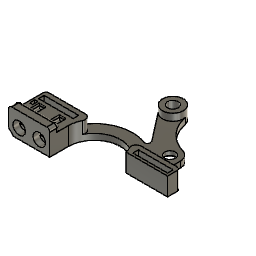
D_Prpbe_Mount v6 (Autodesk Fusion 360 design; units mm, degrees)
Autodesk Fusion 360 part; units mm, degrees
sketch "스케치1" plane through (0, 0, 0) normal (0, 0, 1) x (1, 0, 0)
  circle A0 centre (0, 0) radius 3.675
  circle A1 centre (17.5, -18.9) radius 3.675
  line L0 (30.625, -30.525) -> (30.625, -33.275)
  line L1 (30.625, -33.275) -> (13.375, -33.275)
  line L2 (13.375, -33.275) -> (13.375, -30.525)
  line L3 (-33.625, -33.275) -> (-16.375, -33.275)
  line L4 (-16.375, -33.275) -> (-16.375, -30.525)
  line L5 (-33.625, -30.525) -> (-33.625, -33.275)
  line L6 (-35, -28.225) -> (-18.0402, -28.225)
  line L7 (-14.55, -37.575) -> (-14.55, -46.814)
  line L8 (-14.55, -46.814) -> (-35, -46.814)
  line L9 (-35, -46.814) -> (-35, -28.225)
  line L10 (22.675, -28.225) -> (31.925, -28.225)
  line L11 (31.925, -28.225) -> (31.925, -34.575)
  line L12 (31.925, -34.575) -> (11.2005, -34.575)
  line L13 (22.675, -18.9) -> (22.675, -28.225)
  arc A2 (5.0614, 1.0785) -> (18.9641, -13.9364) centre (24.6222, 5.2465) ccw
  arc A3 (22.675, -18.9) -> (18.9641, -13.9364) centre (17.5, -18.9) ccw
  line L14 (-1.5, -27.846) -> (-1.5, -47.304)
  arc A4 (5.2755, -19.8242) -> (-18.0402, -28.225) centre (-1.5, -37.575) ccw
  line L15 (6.9969, -17.5051) -> (13.5292, -25.9507) construction
  arc A5 (5.0614, 1.0785) -> (-4.0935, -3.1661) centre (0, 0) ccw
  arc A6 (11.2005, -34.575) -> (-14.55, -37.575) centre (-1.5, -37.575) ccw
  arc A7 (13.5292, -25.9507) -> (5.2755, -19.8242) centre (-1.5, -37.575) ccw construction
  line L16 (-4.0935, -3.1661) -> (6.9969, -17.5051)
  arc A8 (5.2755, -19.8242) -> (6.9969, -17.5051) centre (5.8104, -18.4228) ccw
  arc A9 (-4.0935, -3.1661) -> (5.0614, 1.0785) centre (0, 0) ccw
  circle A10 centre (0, 0) radius 2.675
  circle A11 centre (17.5, -18.9) radius 2.675
  line L17 (-18.0402, -28.225) -> (-10.6038, -28.225)
  line L18 (22.675, -28.225) -> (7.6038, -28.225)
  line L19 (13.375, -30.525) -> (30.625, -30.525)
  line L20 (-16.375, -30.525) -> (-33.625, -30.525)
  dimension "d17" = 7.35
  dimension "d18" = 7.35
  dimension "d19" = 17.5
  dimension "d20" = 18.9
  dimension "d22" = 4.125
  dimension "d23" = 17.25
  dimension "d26" = 17.25
  dimension "d28" = 29.75
  dimension "d32" = 1.375
  dimension "d34" = 1.3
  dimension "d36" = 1.3
  dimension "d47" = 10.35
  dimension "d48" = 10.35
  dimension "d52" = 40
  dimension "d54" = 38
  dimension "d55" = 3
  dimension "d56" = 26.1
  dimension "d62" = 13.539
  dimension "d63" = 3
  dimension "d68" = 5.35
  dimension "d69" = 5.35
  dimension "d79" = 2.75
  dimension "d80" = 6.35
  dimension "d81" = 9.325
  constraint coincident A0.centre A5.centre
  constraint vertical L0
  constraint horizontal L1
  constraint vertical L2
  constraint horizontal L3
  constraint vertical L4
  constraint vertical L5
  constraint collinear L1 L3
  constraint horizontal L6
  constraint vertical L7
  constraint horizontal L8
  constraint vertical L9
  constraint horizontal L10
  constraint vertical L11
  constraint horizontal L12
  constraint vertical L13
  constraint concentric A1 A3
  constraint tangent L13 A3
  constraint tangent A2 A5
  constraint tangent A2 A3
  constraint concentric A4 A6
  constraint perpendicular L10 L14
  constraint coincident A4.centre L14
  constraint midpoint A4.centre L14
  constraint symmetric L2 L4 L14
  constraint tangent L15 A5
  constraint tangent A4 L15
  constraint tangent L7 A6
  constraint tangent L15 A8
  constraint tangent A4 A8
  constraint concentric A4 A7
  constraint tangent A5 L16
  constraint equal A5 A9
  constraint concentric A9 A10
  constraint concentric A1 A11
  constraint coincident A6 L17.end
  constraint parallel L6 L17
  constraint coincident A6 L18.end
  constraint perpendicular L13 L18
  constraint perpendicular L0 L19
  constraint perpendicular L5 L20
  constraint collinear L19 L20
  constraint collinear L17 L18
  measures "d17" diameter of A0
  measures "d18" diameter of A1
  measures "d19" horizontal distance of A0.centre A1.centre
  measures "d20" vertical distance of A0.centre A1.centre
  measures "d22" distance of A1.centre L2
  measures "d23" distance of L0.end L1.end
  measures "d26" distance of L3.start L3.end
  measures "d28" distance of L2 L4
  measures "d32" distance of L5 L9
  measures "d34" distance of L0 L11
  measures "d36" distance of L1 L12
  measures "d47" diameter of A5
  measures "d48" diameter of A3
  measures "d52" diameter of A2
  measures "d54" diameter of A4
  measures "d55" distance of L12 A4.centre
  measures "d56" diameter of A6
  measures "d62" distance of L3 L8
  measures "d63" diameter of A8
  measures "d68" diameter of A10
  measures "d69" diameter of A11
  measures "d79" distance of L1 L19
  measures "d80" distance of L10.end L11.end
  measures "d81" distance of A1.centre L10
extrude "돌출1" add sketch "스케치1" along normal blind 3 contours A0 | A1 | L6 L7 L8 L9 A6 L17 | L13 A2 A3 A4 A6 L16 A8 A9 L17 L18 | L10 L11 L12 A6 L18 | A5 A9
extrude "돌출2" add sketch "스케치1" along normal blind 6.5 contours A0 | A5 A9
extrude "돌출3" cut sketch "스케치1" along normal blind 1 contours A0 | A1
extrude "돌출4" add sketch "스케치1" along normal blind 9 contours L6 L7 L8 L9 A6 L17 | L10 L11 L12 A6 L18
chamfer "모따기1" distance 2 distance2 1.5 1 edges at (22, -30.525, 0) measured on face at (19.125, -30.525, 3)
chamfer "모따기1" distance 2 distance2 1.5 1 edges at (-25, -30.525, 0) measured on face at (-22.125, -30.525, 3)
chamfer "모따기2" distance 2.5 angle 45 1 edges at (-35, -37.5195, 0)
sketch "스케치3" plane through (0, 0, 0) normal (0, 0, -1) x (1, 0, 0)
  line L0 (-32.5, 29.025) -> (-32.5, 28.225)
  line L1 (-32.5, 28.225) -> (-18.0402, 28.225)
  arc A0 (-18.0402, 28.225) -> (5.2755, 19.8242) centre (-1.5, 37.575) ccw
  arc A1 (6.9969, 17.5051) -> (5.2755, 19.8242) centre (5.8104, 18.4228) ccw
  line L2 (6.9969, 17.5051) -> (-4.0935, 3.1661)
  arc A2 (-4.0935, 3.1661) -> (5.0614, -1.0785) centre (0, 0) ccw
  arc A3 (18.9641, 13.9364) -> (5.0614, -1.0785) centre (24.6222, -5.2465) ccw
  arc A4 (18.9641, 13.9364) -> (22.675, 18.9) centre (17.5, 18.9) ccw
  line L3 (22.675, 18.9) -> (22.675, 28.225)
  line L4 (22.675, 28.225) -> (31.925, 28.225)
  line L5 (31.925, 28.225) -> (31.925, 34.575)
  line L6 (31.925, 34.575) -> (11.2005, 34.575)
  arc A5 (-14.55, 37.575) -> (11.2005, 34.575) centre (-1.5, 37.575) ccw
  line L7 (-14.55, 37.575) -> (-14.55, 46.814)
  line L8 (-14.55, 46.814) -> (-32.5, 46.814)
  line L9 (-32.5, 46.814) -> (-32.5, 33.275)
  line L10 (-32.5, 33.275) -> (-16.375, 33.275)
  line L11 (-16.375, 33.275) -> (-16.375, 29.025)
  line L12 (-16.375, 29.025) -> (-32.5, 29.025)
  line L13 (30.625, 33.275) -> (30.625, 29.025)
  line L14 (30.625, 29.025) -> (13.375, 29.025)
  line L15 (13.375, 29.025) -> (13.375, 33.275)
  line L16 (13.375, 33.275) -> (30.625, 33.275)
  circle A6 centre (0, 0) radius 3.675
  circle A7 centre (17.5, 18.9) radius 3.675
  line L17 (-32.5, 34.775) -> (-34, 34.775)
  line L18 (-34, 34.775) -> (-34, 37.275)
  line L19 (-34, 37.275) -> (-32.5, 37.275)
  line L20 (-32.5, 37.275) -> (-32.5, 34.775)
  line L21 (-32.5, 39.775) -> (-34, 39.775)
  line L22 (-34, 39.775) -> (-34, 42.275)
  line L23 (-34, 42.275) -> (-32.5, 42.275)
  line L24 (-32.5, 42.275) -> (-32.5, 39.775)
  dimension "d84" = 1.5
  dimension "d85" = 2.5
  dimension "d86" = 1.5
  dimension "d87" = 2.5
  dimension "d88" = 2.5
  constraint horizontal L17
  constraint vertical L18
  constraint horizontal L19
  constraint vertical L20
  constraint coincident L9 L17.start
  constraint horizontal L21
  constraint vertical L22
  constraint horizontal L23
  constraint vertical L24
  constraint coincident L9 L21.start
  constraint collinear L18 L22
  measures "d84" distance of L17.start L17.end
  measures "d85" distance of L17.end L18.end
  measures "d86" distance of L10 L17
  measures "d87" distance of L19 L21
  measures "d88" distance of L21.end L22.end
extrude "돌출5" cut sketch "스케치3" against normal blind 15 contours L9 L17 L18 L19 L20
extrude "돌출6" cut sketch "스케치3" against normal blind 5.75 contours L9 L21 L22 L23 L24
sketch "스케치4" plane through (-35, 0, 0) normal (-1, 0, 0) x (0, -1, 0)
  line L0 (28.225, 2.5) -> (46.814, 2.5)
  line L1 (46.814, 2.5) -> (46.814, 9)
  line L2 (46.814, 9) -> (28.225, 9)
  line L3 (28.225, 9) -> (28.225, 2.5)
  line L4 (34.775, 4.25) -> (37.275, 4.25)
  line L5 (37.275, 4.25) -> (37.275, 5.75)
  line L6 (37.275, 5.75) -> (34.775, 5.75)
  line L7 (34.775, 5.75) -> (34.775, 4.25)
  line L8 (39.775, 4.25) -> (42.275, 4.25)
  line L9 (42.275, 4.25) -> (42.275, 5.75)
  line L10 (42.275, 5.75) -> (39.775, 5.75)
  line L11 (39.775, 5.75) -> (39.775, 4.25)
  line L12 (39.775, 0) -> (39.775, 1.5)
  line L13 (34.775, 0) -> (34.775, 1.5)
  line L14 (37.275, 1.5) -> (37.275, 0)
  line L15 (42.275, 1.5) -> (42.275, 0)
  line L16 (39.775, 0) -> (42.275, 0)
  dimension "d93" = 5.75
  dimension "d94" = 1.5
  constraint horizontal L4
  constraint vertical L5
  constraint horizontal L6
  constraint vertical L7
  constraint horizontal L8
  constraint vertical L9
  constraint horizontal L10
  constraint vertical L11
  constraint collinear L11 L12
  constraint collinear L7 L13
  constraint collinear L5 L14
  constraint collinear L9 L15
  constraint collinear L6 L10
  constraint collinear L4 L8
  measures "d93" distance of L10 L16
  measures "d94" distance of L8.end L9.end
extrude "돌출7" cut sketch "스케치4" against normal up to surface (2.5 mm away) contours L4 L5 L6 L7 | L8 L9 L10 L11
fillet "모깎기1" radius 1 1 edges at (-32.5, -41.025, 5.75)
sketch "스케치5" plane through (0, -46.814, 0) normal (0, -1, 0) x (1, 0, 0)
  line L0 (-35, 2.5) -> (-32.5, 0)
  line L1 (-32.5, 0) -> (-14.55, 0)
  line L2 (-14.55, 0) -> (-14.55, 9)
  line L3 (-14.55, 9) -> (-35, 9)
  line L4 (-35, 9) -> (-35, 2.5)
  line L5 (-14.55, 0) -> (-14.55, 12.25)
  line L6 (-14.55, 12.25) -> (-35, 12.25)
  line L7 (-35, 12.25) -> (-35, 2.5)
  line L8 (-32.5, 0) -> (-14.55, 0)
  circle A0 centre (-29.775, 5) radius 3.1
  circle A1 centre (-19.775, 5) radius 3.1
  line L9 (-29.775, 5) -> (-19.775, 5) construction
  line L10 (-24.775, 9.2865) -> (-24.775, 0.7135) construction
  line L11 (-32.7093, 4) -> (-26.8407, 4)
  line L12 (-22.7093, 4) -> (-16.8407, 4)
  line L13 (-26.8407, 4) -> (-24.775, 4) construction
  line L14 (-24.775, 4) -> (-22.7093, 4) construction
  dimension "d99" = 12.25
  dimension "d100" = 6.2
  dimension "d101" = 6.2
  dimension "d102" = 5
  dimension "d106" = 10
  dimension "d111" = 1
  constraint coincident L1.end L2.start
  constraint perpendicular L3 L5
  constraint perpendicular L4 L6
  constraint coincident L0.start L4.end
  constraint perpendicular L6 L7
  constraint coincident L0.end L1.start
  constraint coincident A0.centre L9.start
  constraint coincident A1.centre L9.end
  constraint horizontal L9
  constraint vertical L10
  constraint midpoint L9 L10
  constraint horizontal L11
  constraint coincident A1 L12.end
  constraint coincident A0 L11.start
  constraint coincident A0 L11.end
  constraint coincident L10 L13.end
  constraint coincident A1 L12.start
  constraint horizontal L12
  constraint collinear L11 L12
  constraint horizontal L14
  measures "d99" distance of L6 L8
  measures "d100" diameter of A0
  measures "d101" diameter of A1
  measures "d102" distance of L8 L9
  measures "d106" distance of A0.centre A1.centre
  measures "d111" distance of A0.centre L11
extrude "돌출8" add sketch "스케치5" against normal blind 5 contours L3 L5 L6 L7
extrude "돌출9" cut sketch "스케치5" against normal blind 3.2 contours A0 L11 | A0 L11 | A1 L12 | A1 L12
extrude "돌출10" cut sketch "스케치5" against normal blind 3.7 contours A0 L11 | A1 L12 picked at (-29.1612, 5.4142) picked at (-18.976, 5.7474)
sketch "스케치6" plane through (0, -43.614, 0) normal (0, -1, 0) x (1, 0, 0)
  line L0 (-16.8407, 4) -> (-22.7093, 4)
  arc A0 (-22.7093, 4) -> (-16.8407, 4) centre (-19.775, 5) ccw
  circle A1 centre (-19.775, 8.1) radius 1.25
  circle A2 centre (-29.775, 8.1) radius 1.25
  circle A3 centre (-19.775, 5) radius 3.1
  circle A4 centre (-29.775, 5) radius 3.1
  line L1 (-19.775, 5) -> (-19.775, 8.1)
  line L2 (-29.775, 5) -> (-29.775, 8.1)
  dimension "d114" = 2.5
  dimension "d115" = 2.5
  constraint coincident A1.centre A3
  constraint coincident A2.centre A4
  constraint coincident A0.centre A3.centre
  constraint coincident A1.centre L1.end
  constraint coincident A4.centre L2.start
  constraint coincident A2.centre L2.end
  constraint vertical L1
  constraint vertical L2
  measures "d114" diameter of A1
  measures "d115" diameter of A2
extrude "돌출11" cut sketch "스케치6" against normal blind 8 contours A1 A3 L1 | A1 A3 | A1 A3 L1 | A2 A4 | A2 A4 L2 | A2 A4 L2 picked at (-29.4705, 8.4731)
fillet "모깎기2" radius 0.5 6 edges at (-18.9075, -38.714, 9) (-19.775, -35.614, 9) (-20.6425, -38.714, 9) (-28.9075, -38.714, 9) (-29.775, -35.614, 9) (-30.6425, -38.714, 9)
fillet "모깎기3" radius 2.5 2 edges at (7.6038, -28.225, 6) (-10.6038, -28.225, 6)
fillet "모깎기4" radius 1.5 2 edges at (-35, -28.225, 5.75) (31.925, -28.225, 4.5)
fillet "모깎기4" radius 1.5 5 edges at (-24.775, -41.814, 12.25) (-35, -44.314, 12.25) (-35, -41.814, 10.625) (-14.55, -44.314, 12.25) (-14.55, -41.814, 10.625)
equation "d54 = ( 19 * 2 ) * 1 mm"
equation "d56 = ( 13.05 * 2 ) * 1 mm"
named bodies: "프로브 마운트"
